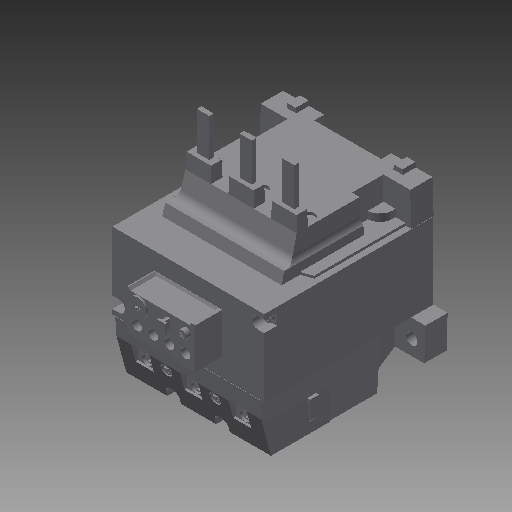
# Autodesk Inventor part: 278463
Saved by Autodesk Inventor 2019.3 (Build 233278000, 278)
## iProperties
Category: PARTsolutions
Company: MOELLER
Created: 2018-10-25
Part Number: 278463
Material: Generic
Catalog Web Link: www.cadenas.de
Description: Bimetal relay ZB up to 150 A-
Vendor: MOELLER
Document SubType Name: Modeling
Designer: psadmin
Manufacturer: MOELLER
Mass: 992.881 g
Surface Area: 1231.4 cm^2
Volume: 992.881 cm^3
Density: 1 g/cm^3
Appearance: PSOLRGB-175-175-175
PSOL_IDENT_0: {$CADENAS_DATA\23d-libs\moeller\2\839\841\844.prj},188 {VTYP=3D},{NB=278463},{LINA=278463},{NN=Bimet
PSOL_IDENT_1: al relay ZB up to 150 A},{DATE=04.10.2018 12:16:44},{GEOMDATE=04.10.2018 08:29:25},{VERSION=v1810040
PSOL_IDENT_2: 82925},{LINEID=370},{WBVAR=},{WBNUMERIC=}  {NB=278463},{LINA=278463},{KT=DUMMY},{PFOTO=2310pic-8.jpg
PSOL_IDENT_3: },{PLID=278463},{DATA_SHEET=Data sheet},{MANUTYPEDESC=ZB150-70},{DESCSHORT=Overload relay, 50-70A, 1
PSOL_IDENT_4: N/O+1N/C},{DESCLONG=Overload relay for direct mounting onto contactor size DILM80 to DILM170, phase
PSOL_IDENT_5: failure sensitivity according to IEC/EN 60947, VDE0660 T.102, suitable for protection of EEX e motor
PSOL_IDENT_6: s, tripping class 10A, screw fixing, Ui 1000V, degree of protection IP00, finger- and back-of-hand p
PSOL_IDENT_7: roof to EN 50274 with vertical actuation from the front, device for world markets, shipping classifi
PSOL_IDENT_8: cation},{EAN=4015082784638},{ECLASS_8_1=27-37-15-01},{PACKAGED_WEIGHT=1.208},{DATA_SHEET_=http://dat
PSOL_IDENT_9: asheet.moeller.net/datasheet.php?model=278463&locale=en_GB},{DATA_SHEET_ENG=http://datasheet.moeller
PSOL_IDENT_10: .net/datasheet.php?model=278463&locale=en_GB},{DATA_SHEET_DEU=http://datasheet.moeller.net/datasheet
PSOL_IDENT_11: .php?model=278463&locale=de_DE}
NN: Bimetal relay ZB up to 150 A
NB: 278463
NBSYN: $PLID.
LINA: 278463
PFOTO: 2310pic-8.jpg
PLID: 278463
DATA_SHEET: Data sheet
MANUTYPEDESC: ZB150-70
DESCSHORT: Overload relay, 50-70A, 1N/O+1N/C
DESCLONG: Overload relay for direct mounting onto contactor size DILM80 to DILM170, phase failure sensitivity according to IEC/EN 60947, VDE0660 T.102, suitable for protection of EEX e motors, tripping class 10A, screw fixing, Ui 1000V, degree of protection IP00, finger- and back-of-hand proof to EN 50274 with vertical actuation from the front, device for world markets, shipping classification
EAN: 4015082784638
ECLASS_8_1: 27-37-15-01
PACKAGED_WEIGHT: 1.208
SUPPLIER: MOELLER
ARTICLENO: 278463
BOMINFO: 278463
CREATOR: CADENAS GmbH
Title: 278463
Author: Cadenas PARTsolutions
Autodesk Inventor part; units mm, degrees
ref_plane "YZ Plane" through (0, 0, 0) normal (1, 0, 0) x (0, 1, 0)
ref_plane "XZ Plane" through (0, 0, 0) normal (0, 1, 0) x (-1, 0, 0)
ref_plane "XY Plane" through (0, 0, 0) normal (0, 0, 1) x (1, 0, 0)
sketch "Sketch_1" plane through (0, 0, 0) normal (1, 0, 0) x (0, 1, 0)
  line L0 (-25, 110.6) -> (-25, 0)
  line L1 (-25, 0) -> (25, 0)
  line L2 (25, 0) -> (25, 110.6)
  line L3 (25, 110.6) -> (-25, 110.6)
  constraints: 8 end point
extrude "Extrusion1" add sketch "Sketch_1" along normal blind 99.6
sketch "Sketch_2" plane through (0, 0, 102.1) normal (0, 0, 1) x (1, 0, 0)
  arc A0 (95.2, 21.8) -> (95.2, 14.2) centre (95.2, 18) ccw
  line L0 (95.2, 14.2) -> (99.6, 14.2)
  line L1 (99.6, 14.2) -> (99.6, 21.8)
  line L2 (99.6, 21.8) -> (95.2, 21.8)
  constraints: 6 end point, 2 point on circle, 1 centre point
extrude "Extrusion2" cut sketch "Sketch_2" along normal blind 10
sketch "Sketch_3" plane through (0, 0, 102.1) normal (0, 0, 1) x (1, 0, 0)
  line L0 (0, -14.2) -> (0, -21.8)
  line L1 (0, -21.8) -> (4.4, -21.8)
  arc A0 (4.4, -21.8) -> (4.4, -14.2) centre (4.4, -18) ccw
  line L2 (4.4, -14.2) -> (0, -14.2)
  constraints: 6 end point, 2 point on circle, 1 centre point
extrude "Extrusion3" cut sketch "Sketch_3" along normal blind 10
sketch "Sketch_4" plane through (0, 0, 102.1) normal (0, 0, 1) x (1, 0, 0)
  circle A0 centre (95.2, 18) radius 3.35
  constraints: 1 centre point
extrude "Extrusion4" add sketch "Sketch_4" along normal blind 2
sketch "Sketch_5" plane through (0, 0, 102.1) normal (0, 0, 1) x (1, 0, 0)
  circle A0 centre (4.4, -18) radius 3.35
  constraints: 1 centre point
extrude "Extrusion5" add sketch "Sketch_5" along normal blind 2
sketch "Sketch_6" plane through (0, 0, 104.1) normal (0, 0, 1) x (1, 0, 0)
  line L0 (92.9614, 18.7151) -> (94.7, 17.7113)
  line L1 (94.7, 17.7113) -> (94.7, 15.7038)
  line L2 (94.7, 15.7038) -> (95.7, 15.7038)
  line L3 (95.7, 15.7038) -> (95.7, 17.7113)
  line L4 (95.7, 17.7113) -> (97.4386, 18.7151)
  line L5 (97.4386, 18.7151) -> (96.9386, 19.5811)
  line L6 (96.9386, 19.5811) -> (95.2, 18.5774)
  line L7 (95.2, 18.5774) -> (93.4614, 19.5811)
  line L8 (93.4614, 19.5811) -> (92.9614, 18.7151)
  constraints: 18 end point
extrude "Extrusion6" cut sketch "Sketch_6" against normal blind 0.95
sketch "Sketch_7" plane through (0, 0, 104.1) normal (0, 0, 1) x (1, 0, 0)
  line L0 (2.1614, -17.2849) -> (3.9, -18.2887)
  line L1 (3.9, -18.2887) -> (3.9, -20.2962)
  line L2 (3.9, -20.2962) -> (4.9, -20.2962)
  line L3 (4.9, -20.2962) -> (4.9, -18.2887)
  line L4 (4.9, -18.2887) -> (6.6386, -17.2849)
  line L5 (6.6386, -17.2849) -> (6.1386, -16.4189)
  line L6 (6.1386, -16.4189) -> (4.4, -17.4226)
  line L7 (4.4, -17.4226) -> (2.6614, -16.4189)
  line L8 (2.6614, -16.4189) -> (2.1614, -17.2849)
  constraints: 18 end point
extrude "Extrusion7" cut sketch "Sketch_7" against normal blind 0.95
sketch "Sketch_8" plane through (0, 0, 128.4) normal (0, 0, 1) x (1, 0, 0)
  line L0 (27.5, -12.7) -> (72.1, -12.7)
  line L1 (72.1, -12.7) -> (72.1, 13.8)
  line L2 (72.1, 13.8) -> (27.5, 13.8)
  line L3 (27.5, 13.8) -> (27.5, -12.7)
  constraints: 8 end point
extrude "Extrusion8" add sketch "Sketch_8" against normal blind 20
sketch "Sketch_9" plane through (0, 0, 128.4) normal (0, 0, 1) x (1, 0, 0)
  line L0 (28.15, 13.8) -> (29.65, 12.3)
  line L1 (29.65, 12.3) -> (68.3, 12.3)
  line L2 (68.3, 12.3) -> (69.8, 13.8)
  line L3 (69.8, 13.8) -> (28.15, 13.8)
  constraints: 8 end point
extrude "Extrusion9" cut sketch "Sketch_9" against normal blind 17.8
sketch "Sketch_10" plane through (27.5, 0, 0) normal (1, 0, 0) x (0, 0, -1)
  line L0 (-111.566, 12.3) -> (-110.6, 12.3)
  line L1 (-110.6, 12.3) -> (-110.6, 13.8)
  line L2 (-110.6, 13.8) -> (-110.7, 13.8)
  line L3 (-110.7, 13.8) -> (-111.566, 12.3)
  constraints: 8 end point
extrude "Extrusion10" add sketch "Sketch_10" along normal blind 44.6
sketch "Sketch_11" plane through (0, 0, 128.4) normal (0, 0, 1) x (1, 0, 0)
  line L0 (63.3, 3.8) -> (66.3, 3.8)
  arc A0 (66.3, 3.8) -> (63.3, 6.8) centre (66.3, 6.8) ccw
  line L1 (63.3, 6.8) -> (63.3, 3.8)
  constraints: 4 end point, 2 point on circle, 1 centre point
extrude "Extrusion11" add sketch "Sketch_11" along normal blind 3
sketch "Sketch_12" plane through (0, 0, 128.4) normal (0, 0, 1) x (1, 0, 0)
  circle A0 centre (35.3, 6.1) radius 6
  constraints: 1 centre point
extrude "Extrusion12" add sketch "Sketch_12" along normal blind 1.3
sketch "Sketch_13" plane through (0, 0, 131.4) normal (0, 0, 1) x (1, 0, 0)
  line L0 (64.5322, 5.7393) -> (65.2393, 5.0322)
  line L1 (65.2393, 5.0322) -> (66.3, 6.0929)
  line L2 (66.3, 6.0929) -> (67.3607, 5.0322)
  line L3 (67.3607, 5.0322) -> (68.0678, 5.7393)
  line L4 (68.0678, 5.7393) -> (67.0071, 6.8)
  line L5 (67.0071, 6.8) -> (68.0678, 7.8607)
  line L6 (68.0678, 7.8607) -> (67.3607, 8.5678)
  line L7 (67.3607, 8.5678) -> (66.3, 7.5071)
  line L8 (66.3, 7.5071) -> (65.2393, 8.5678)
  line L9 (65.2393, 8.5678) -> (64.5322, 7.8607)
  line L10 (64.5322, 7.8607) -> (65.5929, 6.8)
  line L11 (65.5929, 6.8) -> (64.5322, 5.7393)
  constraints: 24 end point
extrude "Extrusion13" cut sketch "Sketch_13" against normal blind 1.69
sketch "Sketch_14" plane through (0, 0, 131.4) normal (0, 0, 1) x (1, 0, 0)
  line L0 (33.4049, 5.6) -> (34.8, 5.6)
  line L1 (34.8, 5.6) -> (34.8, 4.2049)
  line L2 (34.8, 4.2049) -> (35.8, 4.2049)
  line L3 (35.8, 4.2049) -> (35.8, 5.6)
  line L4 (35.8, 5.6) -> (37.1951, 5.6)
  line L5 (37.1951, 5.6) -> (37.1951, 6.6)
  line L6 (37.1951, 6.6) -> (35.8, 6.6)
  line L7 (35.8, 6.6) -> (35.8, 7.9951)
  line L8 (35.8, 7.9951) -> (34.8, 7.9951)
  line L9 (34.8, 7.9951) -> (34.8, 6.6)
  line L10 (34.8, 6.6) -> (33.4049, 6.6)
  line L11 (33.4049, 6.6) -> (33.4049, 5.6)
  constraints: 24 end point
extrude "Extrusion14" cut sketch "Sketch_14" against normal blind 3.2466
sketch "Sketch_15" plane through (0, 3.75, 0) normal (0, 1, 0) x (1, 0, 0)
  line L0 (52.3, -131.9) -> (52.3, -133.4)
  line L1 (52.3, -133.4) -> (57.3, -133.4)
  line L2 (57.3, -133.4) -> (57.3, -131.9)
  line L3 (57.3, -131.9) -> (55.8, -131.9)
  line L4 (55.8, -131.9) -> (55.8, -128.4)
  line L5 (55.8, -128.4) -> (53.8, -128.4)
  line L6 (53.8, -128.4) -> (53.8, -131.9)
  line L7 (53.8, -131.9) -> (52.3, -131.9)
  constraints: 16 end point
extrude "Extrusion15" add sketch "Sketch_15" along normal blind 6
sketch "Sketch_17" plane through (0, 0, 120.2) normal (0, 0, 1) x (1, 0, 0)
  line L0 (29.75, -20.7) -> (69.85, -20.7)
  line L1 (69.85, -20.7) -> (69.85, -0.7)
  line L2 (69.85, -0.7) -> (61.55, -0.7)
  line L3 (61.55, -0.7) -> (61.55, -15.7)
  line L4 (61.55, -15.7) -> (59.25, -15.7)
  line L5 (59.25, -15.7) -> (59.25, -0.7)
  line L6 (59.25, -0.7) -> (50.95, -0.7)
  line L7 (50.95, -0.7) -> (50.95, -15.7)
  line L8 (50.95, -15.7) -> (48.65, -15.7)
  line L9 (48.65, -15.7) -> (48.65, -0.7)
  line L10 (48.65, -0.7) -> (40.35, -0.7)
  line L11 (40.35, -0.7) -> (40.35, -15.7)
  line L12 (40.35, -15.7) -> (38.05, -15.7)
  line L13 (38.05, -15.7) -> (38.05, -0.7)
  line L14 (38.05, -0.7) -> (29.75, -0.7)
  line L15 (29.75, -0.7) -> (29.75, -20.7)
  constraints: 32 end point
extrude "Extrusion16" cut sketch "Sketch_17" against normal blind 3.8
sketch "Sketch_18" plane through (0, 0, 123.15) normal (0, 0, 1) x (1, 0, 0)
  circle A0 centre (33.9, -5.1) radius 3.3
  constraints: 1 centre point
extrude "Extrusion17" cut sketch "Sketch_18" along normal blind 7
sketch "Sketch_19" plane through (0, 0, 123.15) normal (0, 0, 1) x (1, 0, 0)
  circle A0 centre (44.5, -5.1) radius 3.3
  constraints: 1 centre point
extrude "Extrusion18" cut sketch "Sketch_19" along normal blind 7
sketch "Sketch_20" plane through (0, 0, 123.15) normal (0, 0, 1) x (1, 0, 0)
  circle A0 centre (55.1, -5.1) radius 3.3
  constraints: 1 centre point
extrude "Extrusion19" cut sketch "Sketch_20" along normal blind 7
sketch "Sketch_21" plane through (0, 0, 123.15) normal (0, 0, 1) x (1, 0, 0)
  circle A0 centre (65.7, -5.1) radius 3.3
  constraints: 1 centre point
extrude "Extrusion20" cut sketch "Sketch_21" along normal blind 7
sketch "Sketch_22" plane through (0, 0, 123.15) normal (0, 0, 1) x (1, 0, 0)
  circle A0 centre (33.9, -5.1) radius 4.5
  line L0 (31.9, -5.6) -> (33.4, -5.6)
  line L1 (33.4, -5.6) -> (33.4, -9)
  line L2 (33.4, -9) -> (34.4, -9)
  line L3 (34.4, -9) -> (34.4, -5.6)
  line L4 (34.4, -5.6) -> (35.9, -5.6)
  line L5 (35.9, -5.6) -> (35.9, -4.6)
  line L6 (35.9, -4.6) -> (34.4, -4.6)
  line L7 (34.4, -4.6) -> (34.4, -1)
  line L8 (34.4, -1) -> (33.4, -1)
  line L9 (33.4, -1) -> (33.4, -4.6)
  line L10 (33.4, -4.6) -> (31.9, -4.6)
  line L11 (31.9, -4.6) -> (31.9, -5.6)
  constraints: 24 end point, 1 centre point
extrude "Extrusion21" add sketch "Sketch_22" along normal blind 1.2
sketch "Sketch_23" plane through (0, 0, 123.15) normal (0, 0, 1) x (1, 0, 0)
  circle A0 centre (44.5, -5.1) radius 4.5
  line L0 (42.5, -5.6) -> (44, -5.6)
  line L1 (44, -5.6) -> (44, -9)
  line L2 (44, -9) -> (45, -9)
  line L3 (45, -9) -> (45, -5.6)
  line L4 (45, -5.6) -> (46.5, -5.6)
  line L5 (46.5, -5.6) -> (46.5, -4.6)
  line L6 (46.5, -4.6) -> (45, -4.6)
  line L7 (45, -4.6) -> (45, -1)
  line L8 (45, -1) -> (44, -1)
  line L9 (44, -1) -> (44, -4.6)
  line L10 (44, -4.6) -> (42.5, -4.6)
  line L11 (42.5, -4.6) -> (42.5, -5.6)
  constraints: 24 end point, 1 centre point
extrude "Extrusion22" add sketch "Sketch_23" along normal blind 1.2
sketch "Sketch_24" plane through (0, 0, 123.15) normal (0, 0, 1) x (1, 0, 0)
  circle A0 centre (55.1, -5.1) radius 4.5
  line L0 (53.1, -5.6) -> (54.6, -5.6)
  line L1 (54.6, -5.6) -> (54.6, -9)
  line L2 (54.6, -9) -> (55.6, -9)
  line L3 (55.6, -9) -> (55.6, -5.6)
  line L4 (55.6, -5.6) -> (57.1, -5.6)
  line L5 (57.1, -5.6) -> (57.1, -4.6)
  line L6 (57.1, -4.6) -> (55.6, -4.6)
  line L7 (55.6, -4.6) -> (55.6, -1)
  line L8 (55.6, -1) -> (54.6, -1)
  line L9 (54.6, -1) -> (54.6, -4.6)
  line L10 (54.6, -4.6) -> (53.1, -4.6)
  line L11 (53.1, -4.6) -> (53.1, -5.6)
  constraints: 24 end point, 1 centre point
extrude "Extrusion23" add sketch "Sketch_24" along normal blind 1.2
sketch "Sketch_25" plane through (0, 0, 123.15) normal (0, 0, 1) x (1, 0, 0)
  circle A0 centre (65.7, -5.1) radius 4.5
  line L0 (63.7, -5.6) -> (65.2, -5.6)
  line L1 (65.2, -5.6) -> (65.2, -9)
  line L2 (65.2, -9) -> (66.2, -9)
  line L3 (66.2, -9) -> (66.2, -5.6)
  line L4 (66.2, -5.6) -> (67.7, -5.6)
  line L5 (67.7, -5.6) -> (67.7, -4.6)
  line L6 (67.7, -4.6) -> (66.2, -4.6)
  line L7 (66.2, -4.6) -> (66.2, -1)
  line L8 (66.2, -1) -> (65.2, -1)
  line L9 (65.2, -1) -> (65.2, -4.6)
  line L10 (65.2, -4.6) -> (63.7, -4.6)
  line L11 (63.7, -4.6) -> (63.7, -5.6)
  constraints: 24 end point, 1 centre point
extrude "Extrusion24" add sketch "Sketch_25" along normal blind 1.2
sketch "Sketch_26" plane through (0, 0, 123.15) normal (0, 0, 1) x (1, 0, 0)
  circle A0 centre (33.9, -5.1) radius 1.627
  constraints: 1 centre point
extrude "Extrusion25" add sketch "Sketch_26" against normal blind 7
sketch "Sketch_27" plane through (0, 0, 123.15) normal (0, 0, 1) x (1, 0, 0)
  circle A0 centre (44.5, -5.1) radius 1.627
  constraints: 1 centre point
extrude "Extrusion26" add sketch "Sketch_27" against normal blind 7
sketch "Sketch_28" plane through (0, 0, 123.15) normal (0, 0, 1) x (1, 0, 0)
  circle A0 centre (55.1, -5.1) radius 1.627
  constraints: 1 centre point
extrude "Extrusion27" add sketch "Sketch_28" against normal blind 7
sketch "Sketch_29" plane through (0, 0, 123.15) normal (0, 0, 1) x (1, 0, 0)
  circle A0 centre (65.7, -5.1) radius 1.627
  constraints: 1 centre point
extrude "Extrusion28" add sketch "Sketch_29" against normal blind 7
sketch "Sketch_30" plane through (0, 0, 110.6) normal (0, 0, 1) x (1, 0, 0)
  line L0 (39.05, -20) -> (40.28, -25)
  line L1 (40.28, -25) -> (44.82, -25)
  line L2 (44.82, -25) -> (46.05, -20)
  line L3 (46.05, -20) -> (46.05, -12.7)
  line L4 (46.05, -12.7) -> (39.05, -12.7)
  line L5 (39.05, -12.7) -> (39.05, -20)
  constraints: 12 end point
extrude "Extrusion29" cut sketch "Sketch_30" against normal blind 4.4
sketch "Sketch_31" plane through (0, 0, 110.6) normal (0, 0, 1) x (1, 0, 0)
  line L0 (53.55, -20) -> (54.78, -25)
  line L1 (54.78, -25) -> (59.32, -25)
  line L2 (59.32, -25) -> (60.55, -20)
  line L3 (60.55, -20) -> (60.55, -12.7)
  line L4 (60.55, -12.7) -> (53.55, -12.7)
  line L5 (53.55, -12.7) -> (53.55, -20)
  constraints: 12 end point
extrude "Extrusion30" cut sketch "Sketch_31" against normal blind 4.4
sketch "Sketch_32" plane through (0, 0, 110.6) normal (0, 0, 1) x (1, 0, 0)
  line L0 (39.4091, -12.7) -> (39.5518, -16.7876)
  arc A0 (39.5518, -16.7876) -> (40.55, -18.919) centre (42.55, -16.6829) ccw
  line L1 (40.55, -18.919) -> (40.7275, -24)
  line L2 (40.7275, -24) -> (44.3725, -24)
  line L3 (44.3725, -24) -> (44.55, -18.919)
  arc A1 (44.55, -18.919) -> (45.5482, -16.7876) centre (42.55, -16.6829) ccw
  line L4 (45.5482, -16.7876) -> (45.6909, -12.7)
  line L5 (45.6909, -12.7) -> (39.4091, -12.7)
  constraints: 12 end point, 4 point on circle, 2 centre point
extrude "Extrusion31" add sketch "Sketch_32" against normal blind 4.4
sketch "Sketch_33" plane through (0, 0, 110.6) normal (0, 0, 1) x (1, 0, 0)
  line L0 (53.9091, -12.7) -> (54.0518, -16.7876)
  arc A0 (54.0518, -16.7876) -> (55.05, -18.919) centre (57.05, -16.6829) ccw
  line L1 (55.05, -18.919) -> (55.2275, -24)
  line L2 (55.2275, -24) -> (58.8725, -24)
  line L3 (58.8725, -24) -> (59.05, -18.919)
  arc A1 (59.05, -18.919) -> (60.0482, -16.7876) centre (57.05, -16.6829) ccw
  line L4 (60.0482, -16.7876) -> (60.1909, -12.7)
  line L5 (60.1909, -12.7) -> (53.9091, -12.7)
  constraints: 12 end point, 4 point on circle, 2 centre point
extrude "Extrusion32" add sketch "Sketch_33" against normal blind 4.4
sketch "Sketch33" plane through (0, 0, 110.6) normal (0, 0, 1) x (1, 0, 0)
  point P0 (42.55, -16.6)
hole "Hole1" at (42.55, -16.6, 110.6) direction (0, 0, -1) diameter 3.8 depth 0.39
sketch "Sketch34" plane through (0, 0, 110.6) normal (0, 0, 1) x (1, 0, 0)
  point P0 (57.05, -16.6)
hole "Hole2" at (57.05, -16.6, 110.6) direction (0, 0, -1) diameter 3.8 depth 0.39
sketch "Sketch_36" plane through (0, 0, 110.6) normal (0, 0, 1) x (1, 0, 0)
  line L0 (41.55, -16.85) -> (42.3, -16.85)
  line L1 (42.3, -16.85) -> (42.3, -17.6)
  line L2 (42.3, -17.6) -> (42.8, -17.6)
  line L3 (42.8, -17.6) -> (42.8, -16.85)
  line L4 (42.8, -16.85) -> (43.55, -16.85)
  line L5 (43.55, -16.85) -> (43.55, -16.35)
  line L6 (43.55, -16.35) -> (42.8, -16.35)
  line L7 (42.8, -16.35) -> (42.8, -15.6)
  line L8 (42.8, -15.6) -> (42.3, -15.6)
  line L9 (42.3, -15.6) -> (42.3, -16.35)
  line L10 (42.3, -16.35) -> (41.55, -16.35)
  line L11 (41.55, -16.35) -> (41.55, -16.85)
  constraints: 24 end point
extrude "Extrusion33" cut sketch "Sketch_36" against normal blind 1.34
sketch "Sketch_37" plane through (0, 0, 110.6) normal (0, 0, 1) x (1, 0, 0)
  line L0 (56.05, -16.85) -> (56.8, -16.85)
  line L1 (56.8, -16.85) -> (56.8, -17.6)
  line L2 (56.8, -17.6) -> (57.3, -17.6)
  line L3 (57.3, -17.6) -> (57.3, -16.85)
  line L4 (57.3, -16.85) -> (58.05, -16.85)
  line L5 (58.05, -16.85) -> (58.05, -16.35)
  line L6 (58.05, -16.35) -> (57.3, -16.35)
  line L7 (57.3, -16.35) -> (57.3, -15.6)
  line L8 (57.3, -15.6) -> (56.8, -15.6)
  line L9 (56.8, -15.6) -> (56.8, -16.35)
  line L10 (56.8, -16.35) -> (56.05, -16.35)
  line L11 (56.05, -16.35) -> (56.05, -16.85)
  constraints: 24 end point
extrude "Extrusion34" cut sketch "Sketch_37" against normal blind 1.34
sketch "Sketch_38" plane through (0, 0, 50.5) normal (0, 0, 1) x (1, 0, 0)
  line L0 (12.05, -15.2) -> (12.05, -25.2)
  line L1 (12.05, -25.2) -> (24.05, -25.2)
  line L2 (24.05, -25.2) -> (24.05, -20.2)
  line L3 (24.05, -20.2) -> (44.05, -20.2)
  line L4 (44.05, -20.2) -> (44.05, -25.2)
  line L5 (44.05, -25.2) -> (56.05, -25.2)
  line L6 (56.05, -25.2) -> (56.05, -20.2)
  line L7 (56.05, -20.2) -> (76.05, -20.2)
  line L8 (76.05, -20.2) -> (76.05, -25.2)
  line L9 (76.05, -25.2) -> (88.05, -25.2)
  line L10 (88.05, -25.2) -> (88.05, -15.2)
  line L11 (88.05, -15.2) -> (12.05, -15.2)
  constraints: 24 end point
extrude "Extrusion35" add sketch "Sketch_38" along normal blind 3
sketch "Sketch_39" plane through (1.8, 0, 0) normal (1, 0, 0) x (0, 0, -1)
  line L0 (-110.6, -25.2) -> (-110.2127, -36.2915)
  line L1 (-110.2127, -36.2915) -> (-103.86, -60)
  line L2 (-103.86, -60) -> (-33.5, -60)
  line L3 (-33.5, -60) -> (-14, -47)
  line L4 (-14, -47) -> (0.6, -47)
  line L5 (0.6, -47) -> (0.6, -25.2)
  line L6 (0.6, -25.2) -> (-110.6, -25.2)
  constraints: 14 end point
extrude "Extrusion36" add sketch "Sketch_39" along normal blind 96
sketch "Sketch_40" plane through (0, 0, -0.6) normal (0, 0, 1) x (1, 0, 0)
  line L0 (-9.2, -25.2) -> (-8.4387, -47)
  line L1 (-8.4387, -47) -> (108.0387, -47)
  line L2 (108.0387, -47) -> (108.8, -25.2)
  line L3 (108.8, -25.2) -> (-9.2, -25.2)
  constraints: 8 end point
extrude "Extrusion37" add sketch "Sketch_40" along normal blind 14.6
sketch "Sketch_41" plane through (1.8, 0, 0) normal (1, 0, 0) x (0, 0, -1)
  line L0 (-33.5, -60) -> (-14, -47)
  line L1 (-14, -47) -> (-14, -26.252)
  line L2 (-14, -26.252) -> (-32.3215, -26.252)
  line L3 (-32.3215, -26.252) -> (-33.5, -60)
  constraints: 8 end point
extrude "Extrusion38" cut sketch "Sketch_41" along normal blind 9.0325
sketch "Sketch_42" plane through (97.8, 0, 0) normal (1, 0, 0) x (0, 0, -1)
  line L0 (-33.5, -60) -> (-14, -47)
  line L1 (-14, -47) -> (-14, -26.252)
  line L2 (-14, -26.252) -> (-32.3215, -26.252)
  line L3 (-32.3215, -26.252) -> (-33.5, -60)
  constraints: 8 end point
extrude "Extrusion39" cut sketch "Sketch_42" against normal blind 9.0325
sketch "Sketch_43" plane through (0, 0, 110.6) normal (0, 0, 1) x (1, 0, 0)
  line L0 (-8.2, -75.2) -> (107.8, -75.2)
  line L1 (107.8, -75.2) -> (107.8, -25.2)
  line L2 (107.8, -25.2) -> (97.8, -25.2)
  line L3 (97.8, -25.2) -> (96.2286, -70.2)
  line L4 (96.2286, -70.2) -> (3.3714, -70.2)
  line L5 (3.3714, -70.2) -> (1.8, -25.2)
  line L6 (1.8, -25.2) -> (-8.2, -25.2)
  line L7 (-8.2, -25.2) -> (-8.2, -75.2)
  constraints: 16 end point
extrude "Extrusion40" cut sketch "Sketch_43" against normal blind 96.6
sketch "Sketch_44" plane through (2.3, 0, 0) normal (1, 0, 0) x (0, 0, -1)
  line L0 (-110.6, -25.2) -> (-110.2127, -36.2915)
  line L1 (-110.2127, -36.2915) -> (-103.86, -60)
  line L2 (-103.86, -60) -> (-64.9, -60)
  line L3 (-64.9, -60) -> (-64.9, -25.2)
  line L4 (-64.9, -25.2) -> (-110.6, -25.2)
  constraints: 10 end point
extrude "Extrusion41" add sketch "Sketch_44" along normal blind 95
sketch "Sketch_45" plane through (0, 0, 77.2) normal (0, 0, 1) x (1, 0, 0)
  line L0 (1.3, -51.7679) -> (2.3, -53.5)
  line L1 (2.3, -53.5) -> (97.3, -53.5)
  line L2 (97.3, -53.5) -> (98.3, -51.7679)
  line L3 (98.3, -51.7679) -> (98.3, -39)
  line L4 (98.3, -39) -> (1.3, -39)
  line L5 (1.3, -39) -> (1.3, -51.7679)
  constraints: 12 end point
extrude "Extrusion42" add sketch "Sketch_45" along normal mid plane 3.5
sketch "Sketch_46" plane through (0, 0, 77.2) normal (0, 0, 1) x (1, 0, 0)
  line L0 (0.3, -42.5) -> (99.3, -42.5)
  line L1 (99.3, -42.5) -> (99.3, -39)
  line L2 (99.3, -39) -> (0.3, -39)
  line L3 (0.3, -39) -> (0.3, -42.5)
  constraints: 8 end point
extrude "Extrusion43" add sketch "Sketch_46" along normal mid plane 6
sketch "Sketch_47" plane through (0, 0, 110.6) normal (0, 0, 1) x (1, 0, 0)
  line L0 (11.8, -47.5) -> (23.8, -47.5)
  line L1 (23.8, -47.5) -> (23.8, -35.6)
  line L2 (23.8, -35.6) -> (11.8, -35.6)
  line L3 (11.8, -35.6) -> (11.8, -47.5)
  constraints: 8 end point
extrude "Extrusion44" cut sketch "Sketch_47" along normal mid plane 10.2
sketch "Sketch_48" plane through (0, 0, 110.6) normal (0, 0, 1) x (1, 0, 0)
  line L0 (43.8, -47.5) -> (55.8, -47.5)
  line L1 (55.8, -47.5) -> (55.8, -35.6)
  line L2 (55.8, -35.6) -> (43.8, -35.6)
  line L3 (43.8, -35.6) -> (43.8, -47.5)
  constraints: 8 end point
extrude "Extrusion45" cut sketch "Sketch_48" along normal mid plane 10.2
sketch "Sketch_49" plane through (0, 0, 110.6) normal (0, 0, 1) x (1, 0, 0)
  line L0 (75.8, -47.5) -> (87.8, -47.5)
  line L1 (87.8, -47.5) -> (87.8, -35.6)
  line L2 (87.8, -35.6) -> (75.8, -35.6)
  line L3 (75.8, -35.6) -> (75.8, -47.5)
  constraints: 8 end point
extrude "Extrusion46" cut sketch "Sketch_49" along normal mid plane 10.2
sketch "Sketch_50" plane through (0, 0, 110.6) normal (0, 0, 1) x (1, 0, 0)
  circle A0 centre (17.8, -44) radius 3.5
  constraints: 1 centre point
extrude "Extrusion47" cut sketch "Sketch_50" along normal mid plane 13.8
sketch "Sketch_51" plane through (0, 0, 110.6) normal (0, 0, 1) x (1, 0, 0)
  circle A0 centre (49.8, -44) radius 3.5
  constraints: 1 centre point
extrude "Extrusion48" cut sketch "Sketch_51" along normal mid plane 13.8
sketch "Sketch_52" plane through (0, 0, 110.6) normal (0, 0, 1) x (1, 0, 0)
  circle A0 centre (81.8, -44) radius 3.5
  constraints: 1 centre point
extrude "Extrusion49" cut sketch "Sketch_52" along normal mid plane 13.8
sketch "Sketch_53" plane through (0, 0, 110.6) normal (0, 0, 1) x (1, 0, 0)
  line L0 (14.9132, -44) -> (16.3566, -46.5)
  line L1 (16.3566, -46.5) -> (19.2434, -46.5)
  line L2 (19.2434, -46.5) -> (20.6868, -44)
  line L3 (20.6868, -44) -> (19.2434, -41.5)
  line L4 (19.2434, -41.5) -> (16.3566, -41.5)
  line L5 (16.3566, -41.5) -> (14.9132, -44)
  constraints: 12 end point
extrude "Extrusion50" cut sketch "Sketch_53" along normal mid plane 21.8
sketch "Sketch_54" plane through (0, 0, 110.6) normal (0, 0, 1) x (1, 0, 0)
  line L0 (46.9132, -44) -> (48.3566, -46.5)
  line L1 (48.3566, -46.5) -> (51.2434, -46.5)
  line L2 (51.2434, -46.5) -> (52.6868, -44)
  line L3 (52.6868, -44) -> (51.2434, -41.5)
  line L4 (51.2434, -41.5) -> (48.3566, -41.5)
  line L5 (48.3566, -41.5) -> (46.9132, -44)
  constraints: 12 end point
extrude "Extrusion51" cut sketch "Sketch_54" along normal mid plane 21.8
sketch "Sketch_55" plane through (0, 0, 110.6) normal (0, 0, 1) x (1, 0, 0)
  line L0 (78.9132, -44) -> (80.3566, -46.5)
  line L1 (80.3566, -46.5) -> (83.2434, -46.5)
  line L2 (83.2434, -46.5) -> (84.6868, -44)
  line L3 (84.6868, -44) -> (83.2434, -41.5)
  line L4 (83.2434, -41.5) -> (80.3566, -41.5)
  line L5 (80.3566, -41.5) -> (78.9132, -44)
  constraints: 12 end point
extrude "Extrusion52" cut sketch "Sketch_55" along normal mid plane 21.8
sketch "Sketch_56" plane through (0, -40.45, 0) normal (0, 1, 0) x (1, 0, 0)
  line L0 (33.8, -110.6) -> (33.8, -105.2)
  line L1 (33.8, -107.7) -> (37.0813, -107.7)
  line L2 (37.0813, -107.7) -> (37.3, -105.2)
  line L3 (37.3, -105.2) -> (37.55, -105.2)
  line L4 (37.55, -105.2) -> (37.55, -110.6)
  line L5 (37.55, -110.6) -> (33.8, -110.6)
  line L6 (33.8, -110.6) -> (33.8, -107.7)
  constraints: 14 end point
revolve "Revolution1" cut sketch "Sketch_56" angle 360 about axis through (33.8, -40.45, 110.6) along (0, 0, 1)
sketch "Sketch_57" plane through (0, -40.45, 0) normal (0, 1, 0) x (1, 0, 0)
  line L0 (65.8, -110.6) -> (65.8, -105.2)
  line L1 (65.8, -107.7) -> (69.0813, -107.7)
  line L2 (69.0813, -107.7) -> (69.3, -105.2)
  line L3 (69.3, -105.2) -> (69.55, -105.2)
  line L4 (69.55, -105.2) -> (69.55, -110.6)
  line L5 (69.55, -110.6) -> (65.8, -110.6)
  line L6 (65.8, -110.6) -> (65.8, -107.7)
  constraints: 14 end point
revolve "Revolution2" cut sketch "Sketch_57" angle 360 about axis through (65.8, -40.45, 110.6) along (0, 0, 1)
sketch "Sketch_58" plane through (0, 0, 110.6) normal (0, 0, 1) x (1, 0, 0)
  line L0 (30.3, -40.95) -> (33.3, -40.95)
  line L1 (33.3, -40.95) -> (33.3, -42.45)
  line L2 (33.3, -42.45) -> (34.3, -42.45)
  line L3 (34.3, -42.45) -> (34.3, -40.95)
  line L4 (34.3, -40.95) -> (37.3, -40.95)
  line L5 (37.3, -40.95) -> (37.3, -39.95)
  line L6 (37.3, -39.95) -> (34.3, -39.95)
  line L7 (34.3, -39.95) -> (34.3, -38.45)
  line L8 (34.3, -38.45) -> (33.3, -38.45)
  line L9 (33.3, -38.45) -> (33.3, -39.95)
  line L10 (33.3, -39.95) -> (30.3, -39.95)
  line L11 (30.3, -39.95) -> (30.3, -40.95)
  constraints: 24 end point
extrude "Extrusion53" cut sketch "Sketch_58" against normal blind 4.1
sketch "Sketch_59" plane through (0, 0, 110.6) normal (0, 0, 1) x (1, 0, 0)
  line L0 (62.3, -40.95) -> (65.3, -40.95)
  line L1 (65.3, -40.95) -> (65.3, -42.45)
  line L2 (65.3, -42.45) -> (66.3, -42.45)
  line L3 (66.3, -42.45) -> (66.3, -40.95)
  line L4 (66.3, -40.95) -> (69.3, -40.95)
  line L5 (69.3, -40.95) -> (69.3, -39.95)
  line L6 (69.3, -39.95) -> (66.3, -39.95)
  line L7 (66.3, -39.95) -> (66.3, -38.45)
  line L8 (66.3, -38.45) -> (65.3, -38.45)
  line L9 (65.3, -38.45) -> (65.3, -39.95)
  line L10 (65.3, -39.95) -> (62.3, -39.95)
  line L11 (62.3, -39.95) -> (62.3, -40.95)
  constraints: 24 end point
extrude "Extrusion54" cut sketch "Sketch_59" against normal blind 4.1
sketch "Sketch_60" plane through (0, 0, 110.6) normal (0, 0, 1) x (1, 0, 0)
  line L0 (29.3, -77) -> (70.3, -77)
  line L1 (70.3, -77) -> (70.3, -57)
  arc A0 (70.3, -57) -> (61.3, -57) centre (65.8, -57) ccw
  line L2 (61.3, -57) -> (61.3, -72)
  line L3 (61.3, -72) -> (38.3, -72)
  line L4 (38.3, -72) -> (38.3, -57)
  arc A1 (38.3, -57) -> (29.3, -57) centre (33.8, -57) ccw
  line L5 (29.3, -57) -> (29.3, -77)
  constraints: 12 end point, 4 point on circle, 2 centre point
extrude "Extrusion55" cut sketch "Sketch_60" against normal blind 100
sketch "Sketch_61" plane through (0, -60, 0) normal (0, 1, 0) x (1, 0, 0)
  line L0 (9.6, -66.7292) -> (17.8, -69.7138)
  line L1 (17.8, -69.7138) -> (26, -66.7292)
  line L2 (26, -66.7292) -> (26, -53.5)
  line L3 (26, -53.5) -> (9.6, -53.5)
  line L4 (9.6, -53.5) -> (9.6, -66.7292)
  constraints: 10 end point
extrude "Extrusion56" cut sketch "Sketch_61" along normal blind 24.4
sketch "Sketch_62" plane through (0, -60, 0) normal (0, 1, 0) x (1, 0, 0)
  line L0 (41.6, -66.7292) -> (49.8, -69.7138)
  line L1 (49.8, -69.7138) -> (58, -66.7292)
  line L2 (58, -66.7292) -> (58, -53.5)
  line L3 (58, -53.5) -> (41.6, -53.5)
  line L4 (41.6, -53.5) -> (41.6, -66.7292)
  constraints: 10 end point
extrude "Extrusion57" cut sketch "Sketch_62" along normal blind 24.4
sketch "Sketch_63" plane through (0, -60, 0) normal (0, 1, 0) x (1, 0, 0)
  line L0 (73.6, -66.7292) -> (81.8, -69.7138)
  line L1 (81.8, -69.7138) -> (90, -66.7292)
  line L2 (90, -66.7292) -> (90, -53.5)
  line L3 (90, -53.5) -> (73.6, -53.5)
  line L4 (73.6, -53.5) -> (73.6, -66.7292)
  constraints: 10 end point
extrude "Extrusion58" cut sketch "Sketch_63" along normal blind 24.4
sketch "Sketch_64" plane through (0, -60, 0) normal (0, 1, 0) x (1, 0, 0)
  line L0 (9.6, -40.0995) -> (9.6, -50.5)
  line L1 (9.6, -50.5) -> (26, -50.5)
  line L2 (26, -50.5) -> (26, -40.0995)
  line L3 (26, -40.0995) -> (17.8, -37.1149)
  line L4 (17.8, -37.1149) -> (9.6, -40.0995)
  constraints: 10 end point
extrude "Extrusion59" cut sketch "Sketch_64" along normal blind 22.4
sketch "Sketch_65" plane through (0, -60, 0) normal (0, 1, 0) x (1, 0, 0)
  line L0 (41.6, -40.0995) -> (41.6, -50.5)
  line L1 (41.6, -50.5) -> (58, -50.5)
  line L2 (58, -50.5) -> (58, -40.0995)
  line L3 (58, -40.0995) -> (49.8, -37.1149)
  line L4 (49.8, -37.1149) -> (41.6, -40.0995)
  constraints: 10 end point
extrude "Extrusion60" cut sketch "Sketch_65" along normal blind 22.4
sketch "Sketch_66" plane through (0, -60, 0) normal (0, 1, 0) x (1, 0, 0)
  line L0 (73.6, -40.0995) -> (73.6, -50.5)
  line L1 (73.6, -50.5) -> (90, -50.5)
  line L2 (90, -50.5) -> (90, -40.0995)
  line L3 (90, -40.0995) -> (81.8, -37.1149)
  line L4 (81.8, -37.1149) -> (73.6, -40.0995)
  constraints: 10 end point
extrude "Extrusion61" cut sketch "Sketch_66" along normal blind 22.4
sketch "Sketch_67" plane through (0, 0, 8) normal (0, 0, 1) x (1, 0, 0)
  line L0 (3.8, 20.2) -> (95.8, 20.2)
  line L1 (95.8, 20.2) -> (95.8, 25.2)
  line L2 (95.8, 25.2) -> (94.8, 25.2)
  line L3 (94.8, 25.2) -> (94.8, 22.2)
  line L4 (94.8, 22.2) -> (4.8, 22.2)
  line L5 (4.8, 22.2) -> (4.8, 25.2)
  line L6 (4.8, 25.2) -> (3.8, 25.2)
  line L7 (3.8, 25.2) -> (3.8, 20.2)
  constraints: 16 end point
extrude "Extrusion62" add sketch "Sketch_67" along normal blind 66
sketch "Sketch_68" plane through (0, 0, 0) normal (1, 0, 0) x (0, 1, 0)
  line L0 (25.2, 88.5957) -> (25.2, -0.6)
  line L1 (25.2, -0.6) -> (47, -0.6)
  line L2 (47, -0.6) -> (47, 68.5)
  line L3 (47, 68.5) -> (66.9878, 69.198)
  line L4 (66.9878, 69.198) -> (66.9878, 75.302)
  line L5 (66.9878, 75.302) -> (47, 76)
  line L6 (47, 76) -> (36.5248, 78.905)
  arc A0 (32.1282, 84.6868) -> (36.5248, 78.905) centre (38.1282, 84.6868) ccw
  line L7 (32.1282, 84.6868) -> (32.1282, 86.6743)
  line L8 (32.1282, 86.6743) -> (25.2, 88.5957)
  constraints: 18 end point, 2 point on circle, 1 centre point
extrude "Extrusion63" add sketch "Sketch_68" along normal blind 99.6
sketch "Sketch_70" plane through (0, 0, 110.6) normal (0, 0, 1) x (1, 0, 0)
  line L0 (-4.4419, 77) -> (-4.4419, 25.2)
  line L1 (-4.4419, 25.2) -> (10.5581, 25.2)
  line L2 (10.5581, 25.2) -> (10.8, 32.1282)
  arc A0 (10.8, 32.1282) -> (12.9684, 36.5391) centre (6.9721, 36.7485) ccw
  line L3 (12.9684, 36.5391) -> (13.6829, 57)
  line L4 (13.6829, 57) -> (29.8, 57)
  line L5 (29.8, 57) -> (30.1492, 47)
  line L6 (30.1492, 47) -> (41.4554, 47)
  line L7 (41.4554, 47) -> (41.8046, 57)
  line L8 (41.8046, 57) -> (57.7954, 57)
  line L9 (57.7954, 57) -> (58.1446, 47)
  line L10 (58.1446, 47) -> (69.4508, 47)
  line L11 (69.4508, 47) -> (69.8, 57)
  line L12 (69.8, 57) -> (85.9171, 57)
  line L13 (85.9171, 57) -> (86.6316, 36.5391)
  arc A1 (86.6316, 36.5391) -> (88.8, 32.1282) centre (92.6279, 36.7485) ccw
  line L14 (88.8, 32.1282) -> (89.0419, 25.2)
  line L15 (89.0419, 25.2) -> (104.0419, 25.2)
  line L16 (104.0419, 25.2) -> (104.0419, 77)
  line L17 (104.0419, 77) -> (-4.4419, 77)
  constraints: 36 end point, 4 point on circle, 2 centre point
extrude "Extrusion64" cut sketch "Sketch_70" against normal blind 96.5738
sketch "Sketch_69" plane through (0, 26.7, 0) normal (0, 1, 0) x (1, 0, 0)
  line L0 (3.8, -74.1307) -> (17.5374, -79.1307)
  line L1 (17.5374, -79.1307) -> (82.0626, -79.1307)
  line L2 (82.0626, -79.1307) -> (95.8, -74.1307)
  line L3 (95.8, -74.1307) -> (95.8, 0)
  line L4 (95.8, 0) -> (3.8, 0)
  line L5 (3.8, 0) -> (3.8, -74.1307)
  constraints: 12 end point
extrude "Extrusion65" add sketch "Sketch_69" against normal blind 1.5
sketch "Sketch_71" plane through (0, 26.7, 0) normal (0, 1, 0) x (1, 0, 0)
  line L0 (-1.7, -34.6752) -> (18.3, -34.6752)
  line L1 (18.3, -34.6752) -> (18.3, -14.0262)
  line L2 (18.3, -14.0262) -> (-1.7, -14.0262)
  line L3 (-1.7, -14.0262) -> (-1.7, -34.6752)
  constraints: 8 end point
extrude "Extrusion66" cut sketch "Sketch_71" along normal blind 30
sketch "Sketch_72" plane through (0, 26.7, 0) normal (0, 1, 0) x (1, 0, 0)
  line L0 (81.3, -34.6752) -> (101.3, -34.6752)
  line L1 (101.3, -34.6752) -> (101.3, -14.0262)
  line L2 (101.3, -14.0262) -> (81.3, -14.0262)
  line L3 (81.3, -14.0262) -> (81.3, -34.6752)
  constraints: 8 end point
extrude "Extrusion67" cut sketch "Sketch_72" along normal blind 30
sketch "Sketch_89" plane through (0, 0, 0) normal (0, 0, 1) x (1, 0, 0)
  line L0 (0, 25.2) -> (0.873, 50.2)
  line L1 (0.873, 50.2) -> (98.727, 50.2)
  line L2 (98.727, 50.2) -> (99.6, 25.2)
  line L3 (99.6, 25.2) -> (99.6, 55.2)
  line L4 (99.6, 55.2) -> (0, 55.2)
  line L5 (0, 55.2) -> (0, 25.2)
  constraints: 12 end point
extrude "Extrusion68" cut sketch "Sketch_89" along normal mid plane 40
sketch "Sketch_73" plane through (0, 26.7, 0) normal (0, 1, 0) x (1, 0, 0)
  line L0 (10.3338, -7.5316) -> (10.3338, -16)
  arc A0 (10.3338, -16) -> (18.8022, -7.5316) centre (18.8022, -16) ccw
  line L1 (18.8022, -7.5316) -> (10.3338, -7.5316)
  constraints: 4 end point, 2 point on circle, 1 centre point
extrude "Extrusion69" add sketch "Sketch_73" along normal blind 4.8
sketch "Sketch_74" plane through (0, 26.7, 0) normal (0, 1, 0) x (1, 0, 0)
  arc A0 (80.7978, -7.5316) -> (89.2662, -16) centre (80.7978, -16) ccw
  line L0 (89.2662, -16) -> (89.2662, -7.5316)
  line L1 (89.2662, -7.5316) -> (80.7978, -7.5316)
  constraints: 4 end point, 2 point on circle, 1 centre point
extrude "Extrusion70" add sketch "Sketch_74" along normal blind 4.8
sketch "Sketch_75" plane through (0, 0, -0.6) normal (0, 0, 1) x (1, 0, 0)
  line L0 (10.6602, 35) -> (88.9399, 35)
  line L1 (88.9399, 35) -> (87.6276, 50)
  line L2 (87.6276, 50) -> (81.9725, 50)
  line L3 (81.9725, 50) -> (80.9226, 38)
  line L4 (80.9226, 38) -> (18.6775, 38)
  line L5 (18.6775, 38) -> (17.6276, 50)
  line L6 (17.6276, 50) -> (11.9725, 50)
  line L7 (11.9725, 50) -> (10.6602, 35)
  constraints: 16 end point
extrude "Extrusion71" add sketch "Sketch_75" along normal blind 8.5514
sketch "Sketch_76" plane through (0, 0, 70) normal (0, 0, 1) x (1, 0, 0)
  line L0 (17.8, 37) -> (81.8, 37)
  line L1 (81.8, 37) -> (81.8, 82)
  line L2 (81.8, 82) -> (73.8, 82)
  line L3 (73.8, 82) -> (73.8, 42)
  line L4 (73.8, 42) -> (53.8, 42)
  line L5 (53.8, 42) -> (53.8, 82)
  line L6 (53.8, 82) -> (45.8, 82)
  line L7 (45.8, 82) -> (45.8, 42)
  line L8 (45.8, 42) -> (25.8, 42)
  line L9 (25.8, 42) -> (25.8, 82)
  line L10 (25.8, 82) -> (17.8, 82)
  line L11 (17.8, 82) -> (17.8, 37)
  constraints: 24 end point
extrude "Extrusion72" add sketch "Sketch_76" along normal blind 3
sketch "Sketch_77" plane through (0, 0, -0.6) normal (0, 0, 1) x (1, 0, 0)
  line L0 (27.8, 35.5) -> (71.8, 35.5)
  line L1 (71.8, 35.5) -> (71.8, 47)
  line L2 (71.8, 47) -> (27.8, 47)
  line L3 (27.8, 47) -> (27.8, 35.5)
  constraints: 8 end point
extrude "Extrusion73" cut sketch "Sketch_77" along normal blind 6.6
sketch "Sketch78" plane through (13.3337, 47, 68.5) normal (0, 1, 0) x (1, 0, 0)
  point P0 (5.4663, 6.5)
hole "Hole3" at (18.8, 47, 62) direction (0, -1, 0) diameter 7 depth 1.8
sketch "Sketch79" plane through (13.3337, 47, 68.5) normal (0, 1, 0) x (1, 0, 0)
  point P0 (36.4663, 6.5)
hole "Hole4" at (49.8, 47, 62) direction (0, -1, 0) diameter 7 depth 1.8
sketch "Sketch80" plane through (13.3337, 47, 68.5) normal (0, 1, 0) x (1, 0, 0)
  point P0 (67.4663, 6.5)
hole "Hole5" at (80.8, 47, 62) direction (0, -1, 0) diameter 7 depth 1.8
sketch "Sketch_81" plane through (0, 0, 0) normal (0, 0, 1) x (1, 0, 0)
  circle A0 centre (9.8, 37) radius 5
  constraints: 1 centre point
extrude "Extrusion74" add sketch "Sketch_81" against normal blind 1
sketch "Sketch_82" plane through (0, 0, 0) normal (0, 0, 1) x (1, 0, 0)
  circle A0 centre (89.8, 37) radius 5
  constraints: 1 centre point
extrude "Extrusion75" add sketch "Sketch_82" against normal blind 1
sketch "Sketch_83" plane through (0, 0, 0) normal (0, 0, 1) x (1, 0, 0)
  circle A0 centre (-0.2, -37) radius 5.8
  constraints: 1 centre point
extrude "Extrusion76" add sketch "Sketch_83" against normal blind 1
sketch "Sketch_84" plane through (0, 0, 0) normal (0, 0, 1) x (1, 0, 0)
  circle A0 centre (99.8, -37) radius 5.8
  constraints: 1 centre point
extrude "Extrusion77" add sketch "Sketch_84" against normal blind 1
sketch "Sketch_85" plane through (0, 0, 0) normal (0, 0, 1) x (1, 0, 0)
  circle A0 centre (9.8, 37) radius 3.5
  constraints: 1 centre point
extrude "Extrusion78" cut sketch "Sketch_85" along normal mid plane 25.58
sketch "Sketch_86" plane through (0, 0, 0) normal (0, 0, 1) x (1, 0, 0)
  circle A0 centre (89.8, 37) radius 3.5
  constraints: 1 centre point
extrude "Extrusion79" cut sketch "Sketch_86" along normal mid plane 25.58
sketch "Sketch_87" plane through (0, 0, 0) normal (0, 0, 1) x (1, 0, 0)
  circle A0 centre (-0.2, -37) radius 3.8
  constraints: 1 centre point
extrude "Extrusion80" cut sketch "Sketch_87" along normal mid plane 30
sketch "Sketch_88" plane through (0, 0, 0) normal (0, 0, 1) x (1, 0, 0)
  circle A0 centre (99.8, -37) radius 3.8
  constraints: 1 centre point
extrude "Extrusion81" cut sketch "Sketch_88" along normal mid plane 30
sketch "Sketch_90" plane through (0, -12.7, 0) normal (0, 1, 0) x (1, 0, 0)
  line L0 (52.2, -133.2) -> (58, -133.2)
  line L1 (58, -133.2) -> (58, -123.2)
  line L2 (58, -123.2) -> (52.2, -123.2)
  line L3 (52.2, -123.2) -> (52.2, -133.2)
  constraints: 8 end point
extrude "Extrusion82" cut sketch "Sketch_90" along normal blind 1.8
body "Solid1"
